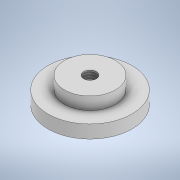
# Autodesk Inventor part: knurledKnob
Saved by Autodesk Inventor 2021 (Build 250183000, 183)
## iProperties
Created: 2020-07-17
Part Number: knurledKnob
Material: Generic
Document SubType Name: Modeling
Designer: robst
Density: 1 g/cm^3
Appearance: Default
Author: robst
Autodesk Inventor part; units mm, degrees
ref_plane "YZ Plane" through (0, 0, 0) normal (1, 0, 0) x (0, 1, 0)
ref_plane "XZ Plane" through (0, 0, 0) normal (0, 1, 0) x (-1, 0, 0)
ref_plane "XY Plane" through (0, 0, 0) normal (0, 0, 1) x (1, 0, 0)
sketch "Sketch1" plane through (0, 0, 0) normal (0, 1, 0) x (-1, 0, 0)
  circle A0 centre (0, 0) radius 13.081
  dimension "outerDiamKnurledKnob" = 26.162
  constraints: 1 centre point, 1 coincident
  measures "outerDiamKnurledKnob" diameter of A0
extrude "Extrusion1" add sketch "Sketch1" along normal blind 4.064
sketch "Sketch2" plane through (0, 4.064, 0) normal (0, 1, 0) x (1, 0, 0)
  circle A0 centre (0, 0) radius 7.9375
  dimension "innerRingDiam" = 15.875
  constraints: 1 centre point, 1 coincident
  measures "innerRingDiam" diameter of A0
extrude "Extrusion2" add sketch "Sketch2" along normal blind 3.937
sketch "Sketch3" plane through (0, 8.001, 0) normal (0, 1, 0) x (1, 0, 0)
  point P0 (0, 0)
  point P1 (0, 0)
  constraints: 1 coincident
hole "Hole1" at (0, 8.001, 0) direction (0, -1, 0) diameter 3.9624 depth 6.35 thread size "10-32 UNF" class "2B" standard "ANSI Unified Screw Threads"
body "Solid1"
